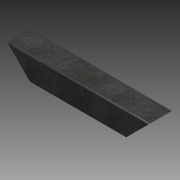
# Autodesk Inventor part: 45degree_brace
Saved by Autodesk Inventor 2015 SP1 (Build 190203100, 203)
## iProperties
Created: 2016-02-03
Part Number: 45degree_brace
Material: Steel
Document SubType Name: Modeling
Designer: guillemd
Density: 7.85 g/cm^3
Appearance: Plate
Mass: 1923.5 g
Surface Area: 2349.41 cm^2
Volume: 245.032 cm^3
Author: guillemd
Autodesk Inventor part; units mm, degrees
ref_plane "YZ Plane" through (0, 0, 0) normal (1, 0, 0) x (0, 1, 0)
ref_plane "XZ Plane" through (0, 0, 0) normal (0, 1, 0) x (-1, 0, 0)
ref_plane "XY Plane" through (0, 0, 0) normal (0, 0, 1) x (1, 0, 0)
sketch "Sketch1" plane through (0, 0, 0) normal (1, 0, 0) x (0, 1, 0)
  line L0 (25.4, 25.4) -> (-25.4, 25.4)
  line L1 (-25.4, 25.4) -> (-25.4, -25.4)
  line L2 (-25.4, -25.4) -> (25.4, -25.4)
  line L3 (25.4, -25.4) -> (25.4, 25.4)
  line L4 (23.2918, 23.2918) -> (-23.2918, 23.2918)
  line L5 (-23.2918, 23.2918) -> (-23.2918, -23.2918)
  line L6 (-23.2918, -23.2918) -> (23.2918, -23.2918)
  line L7 (23.2918, -23.2918) -> (23.2918, 23.2918)
  point P0 (0, 0)
  point P1 (0, -25.4)
  point P2 (25.4, 0)
  dimension "d0" = 50.8
  dimension "d1" = 50.8
  dimension "d2" = 2.1082
  constraints: 16 end point, 4 parallel, 2 midpoint, 2 perpendicular, 1 horizontal, 1 horizontal alignment, 1 vertical alignment, 3 other
  measures "d0" distance of L1.end L2.end
  measures "d1" distance of L2.end L0.start
  measures "d2" distance between parallel lines of L3 L7
extrude "Extrusion1" add sketch "Sketch1" along normal blind 304.8
fillet "Fillet1" radius 3.175 4 edges at (152.4, 25.4, 25.4) (152.4, -25.4, 25.4) (152.4, 25.4, -25.4) (152.4, -25.4, -25.4)
sketch "Sketch2" plane through (0, -22.225, 25.4) normal (0, 0, 1) x (1, 0, 0)
  line L0 (0, 44.45) -> (0, 0) projected
  line L1 (304.8, 44.45) -> (304.8, 0) projected
  line L2 (0, -3.175) -> (0, 47.625)
  line L3 (0, 45.5168) -> (0, -1.0668) projected
  line L4 (0, 47.625) -> (50.8, -3.175)
  line L5 (0, -3.175) -> (50.8, -3.175)
  line L6 (304.8, -3.175) -> (304.8, 47.625)
  line L7 (304.8, 47.625) -> (254, -3.175)
  line L8 (254, -3.175) -> (304.8, -3.175)
  line L9 (0, -3.175) -> (304.8, -3.175) projected
  point P0 (0, 22.225)
  dimension "d6" = 45
  dimension "d7" = 45
  constraints: 12 end point, 2 point on line, 1 collinear
  measures "d6" angle of L0 L4
  measures "d7" angle of L1 L7
extrude "Extrusion2" cut sketch "Sketch2" against normal through all
body "Solid1"
